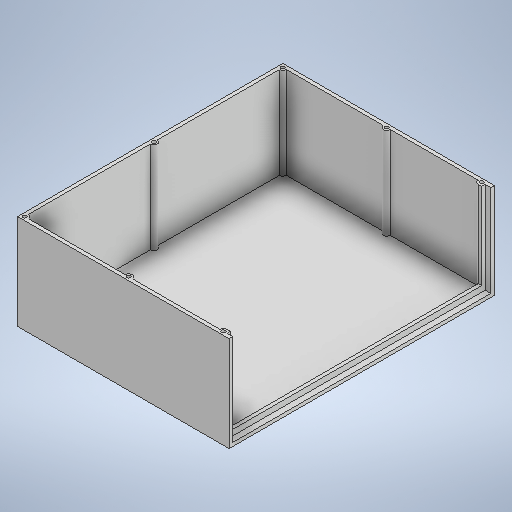
# Autodesk Inventor part: controller-base
Saved by Autodesk Inventor 2025.2 (Build 292293000, 293)
## iProperties
Created: 2025-04-21
Part Number: controller-base
Material: Generic
Document SubType Name: Modeling
Designer: tdeboutte
Density: 1 g/cm^3
Appearance: Default
Author: tdeboutte
Autodesk Inventor part; units mm, degrees
ref_plane "YZ Plane" through (0, 0, 0) normal (1, 0, 0) x (0, 1, 0)
ref_plane "XZ Plane" through (0, 0, 0) normal (0, 1, 0) x (-1, 0, 0)
ref_plane "XY Plane" through (0, 0, 0) normal (0, 0, 1) x (1, 0, 0)
sketch "Sketch1" plane through (0, 0, 0) normal (0, 1, 0) x (-1, 0, 0)
  line L0 (0, 0) -> (120, 0)
  line L1 (120, 0) -> (120, -150.5)
  line L2 (120, -150.5) -> (0, -150.5)
  line L3 (0, -150.5) -> (0, 0)
  line L4 (118, -148.5) -> (118, -2)
  line L5 (118, -2) -> (2, -2)
  line L6 (0, -148.5) -> (118, -148.5)
  line L7 (2, -2) -> (0, -2)
  line L8 (1.5, -2) -> (1.5, -148.5)
  point P0 (0, -144.5)
  dimension "d0" = 150.5
  dimension "d1" = 120
  dimension "d2" = 2
  dimension "d3" = 1.5
  dimension "d13" = 2
  dimension "d14" = 2
  constraints: 18 end point, 4 perpendicular, 4 point on line, 3 parallel, 1 horizontal, 1 other
  measures "d0" distance of L2.end L0.start
  measures "d1" distance of L1.end L2.end
  measures "d2" distance between parallel lines of L1 L4
  measures "d3" distance between parallel lines of L3 L8
  measures "d13" distance between parallel lines of L2 L6
  measures "d14" distance between parallel lines of L0 L5
extrude "Extrusion1" add sketch "Sketch1" along normal blind 52 contours L0 L1 L2 L3 L6 L4 L5 L7
sketch "Sketch2" plane through (0, 0, 0) normal (0, -1, 0) x (1, 0, 0)
  line L0 (-120, -150.5) -> (-120, 0) projected
  line L1 (0, -150.5) -> (-120, -150.5) projected
  line L2 (0, -148.5) -> (0, -150.5) projected
  line L3 (-118, -148.5) -> (0, -148.5) projected
  line L4 (0, 0) -> (0, -2) projected
  line L5 (-120, 0) -> (0, 0) projected
  line L6 (0, -150.5) -> (-120, -150.5)
  line L7 (-120, -150.5) -> (-120, 0)
  line L8 (-120, 0) -> (0, 0)
  line L9 (0, 0) -> (0, -150.5)
  line L10 (-118, -2) -> (-118, -148.5) projected
  line L11 (0, -2) -> (-118, -2) projected
  constraints: 8 end point, 2 parallel, 1 horizontal, 1 perpendicular
extrude "Extrusion2" add sketch "Sketch2" along normal blind 2
sketch "Sketch3" plane through (0, 0, 0) normal (0, 1, 0) x (1, 0, 0)
  line L0 (0, 2) -> (-118, 2) projected
  line L1 (0, 148.5) -> (0, 2) projected
  line L2 (-118, 148.5) -> (0, 148.5) projected
  line L3 (-118, 2) -> (-118, 148.5) projected
  line L4 (-3.2, 2) -> (-3.2, 148.5)
  circle A0 centre (-118, 2) radius 2
  line L5 (-120, 0) -> (-120, 150.5) projected
  circle A1 centre (-118, 148.5) radius 2
  circle A2 centre (-5.2, 2) radius 2
  line L6 (-120, 0) -> (0, 0) projected
  line L7 (-5.2, 4) -> (-3.2, 4)
  circle A3 centre (-5.2, 148.5) radius 2
  line L8 (-5.2, 146.5) -> (-3.2, 146.5)
  circle A4 centre (-118, 75.25) radius 2
  circle A5 centre (-59, 2) radius 2
  circle A6 centre (-59, 148.5) radius 2
  line L9 (0, 150.5) -> (-120, 150.5) projected
  point P0 (-7.2, 148.5)
  point P1 (-3.2, 146.5)
  point P2 (-3.2, 148.5)
  point P3 (-7.2, 2)
  point P4 (-57, 148.5)
  point P5 (-61, 148.5)
  point P6 (-118, 146.5)
  point P7 (-116, 148.5)
  point P8 (-116, 2)
  point P9 (-118, 4)
  point P10 (-118, 73.25)
  point P11 (-118, 77.25)
  dimension "d15" = 3.2
  constraints: 6 end point, 5 centre point, 5 point on line, 3 horizontal, 3 midpoint, 2 coincident, 2 perpendicular, 2 tangent, 1 vertical, 6 other
  measures "d15" distance between parallel lines of L1 L4
extrude "Extrusion3" add sketch "Sketch3" along normal up to surface (52 mm away) contours A2 L0 | A2 L7 L4 | L0 A2 | A3 L2 | L4 L8 A3 | L2 A3 | A5 L0 | L0 A5 | A0 L3 L0 | A6 L2 | L2 A6 | L0 L3 A0 | A1 L2 L3 | A4 L3 | A1 L3 L2 | L3 A4
sketch "Sketch5" plane through (0, 52, 0) normal (0, 1, 0) x (1, 0, 0)
  arc A0 (-5.2, 4) -> (-7.2, 2) centre (-5.2, 2) ccw projected
  arc A1 (-57, 2) -> (-61, 2) centre (-59, 2) ccw projected
  arc A2 (-116, 2) -> (-118, 4) centre (-118, 2) ccw projected
  arc A3 (-118, 73.25) -> (-118, 77.25) centre (-118, 75.25) ccw projected
  arc A4 (-118, 146.5) -> (-116, 148.5) centre (-118, 148.5) ccw projected
  arc A5 (-61, 148.5) -> (-57, 148.5) centre (-59, 148.5) ccw projected
  arc A6 (-7.2, 148.5) -> (-5.2, 146.5) centre (-5.2, 148.5) ccw projected
  point P0 (0, 0)
hole "Hole1" at (-118, 52, -2) at (-118, 52, -75.25) at (-118, 52, -148.5) at (-59, 52, -148.5) at (-5.2, 52, -2) at (-5.2, 52, -148.5) at (-59, 52, -2) direction (0, -1, 0) diameter 2.1 depth 20
sketch "Sketch6" plane through (0, 0, -2) normal (0, 0, -1) x (-1, 0, 0)
  line L0 (5.2, 52) -> (3.2, 52) projected
  line L1 (3.2, 0) -> (3.2, 52) projected
  line L2 (5.2, 0) -> (3.2, 0) projected
  line L3 (5.2, 0) -> (5.2, 52) projected
  line L4 (7.2, 52) -> (7.2, 0) projected
  line L5 (7.2, 52) -> (5.2, 52) projected
  line L6 (5.2, 0) -> (5.2, 52) projected
  line L7 (7.2, 0) -> (5.2, 0) projected
  line L8 (3.2, 0) -> (5.2, 0)
  line L9 (5.2, 0) -> (5.2, 3.2)
  line L10 (5.2, 3.2) -> (3.2, 3.2)
  line L11 (3.2, 3.2) -> (3.2, 0)
  arc A0 (7.2, 0) -> (5.2, 3.2) centre (3.64, 0) ccw
  point P0 (0, 0)
  point P1 (3.2, 3.2)
  dimension "d29" = 3.2
  constraints: 8 end point, 2 parallel, 2 point on circle, 1 centre point, 1 horizontal, 1 perpendicular, 1 point on line, 1 tangent
  measures "d29" distance of L9.end L8.end
extrude "Extrusion5" add sketch "Sketch6" along normal through all contours A0 L7 L3 | L3 L2 L1 L10
equation "\"d13\" = d2"
body "Solid1"
